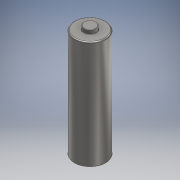
# Autodesk Inventor part: AA_Battery
Saved by Autodesk Inventor 2018 (Build 220112000, 112)
## iProperties
Created: 2019-05-16
Part Number: AA_Battery
Material: 一般
Document SubType Name: Modeling
Designer: ku_sk
Density: 2.40036 g/cm^3
Appearance: 半つや出し
Mass: 18 g
Surface Area: 24.4736 cm^2
Volume: 7.49886 cm^3
Author: ku_sk
Autodesk Inventor part; units mm, degrees
ref_plane "YZ Plane" through (0, 0, 0) normal (1, 0, 0) x (0, 1, 0)
ref_plane "XZ Plane" through (0, 0, 0) normal (0, 1, 0) x (-1, 0, 0)
ref_plane "XY Plane" through (0, 0, 0) normal (0, 0, 1) x (1, 0, 0)
sketch "スケッチ1" plane through (0, 0, 0) normal (0, 0, 1) x (1, 0, 0)
  circle A0 centre (0, 0) radius 7
  dimension "d0" = 14
  constraints: 1 centre point, 1 coincident
  measures "d0" diameter of A0
extrude "押し出し1" add sketch "スケッチ1" along normal mid plane 48.5
sketch "スケッチ2" plane through (0, 0, 24.25) normal (0, 0, 1) x (1, 0, 0)
  circle A0 centre (0, 0) radius 2.65
  dimension "d3" = 5.3
  constraints: 1 centre point, 1 coincident
  measures "d3" diameter of A0
extrude "押し出し2" add sketch "スケッチ2" along normal blind 1.7
fillet "フィレット1" radius 0.5 2 edges at (-7, 0, 24.25) (-7, 0, -24.25)
fillet "フィレット2" radius 0.2 2 edges at (-2.65, 0, 25.95) (-2.65, 0, 24.25)
